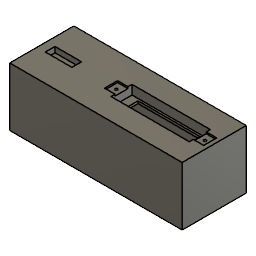
Base Pantalla - Pila T.D.I (Autodesk Fusion 360 design; units mm, degrees)
part number: 2026-07-05-14-44-51-379
Autodesk Fusion 360 part; units mm, degrees
note: some values were not read from the file. Set by a fixed rule: which sketch regions a step uses.
sketch "Boceto1" plane through (0, 0, 0) normal (0, 1, 0) x (1, 0, 0)
  line L0 (0, 0) -> (220, 0)
  line L1 (220, 0) -> (220, 60)
  line L2 (220, 60) -> (0, 60)
  line L3 (0, 60) -> (0, 0)
  line L4 (227, -7) -> (227, 67)
  line L5 (227, 67) -> (-7, 67)
  line L6 (-7, 67) -> (-7, -7)
  line L7 (-7, -7) -> (227, -7)
  line L8 (217, 3) -> (217, 57)
  line L9 (217, 57) -> (3, 57)
  line L10 (3, 57) -> (3, 3)
  line L11 (3, 3) -> (217, 3)
  dimension "d1" = 220
  dimension "d2" = 60
  dimension "d3" = 7
  dimension "d4" = -3
  constraint horizontal L0
  constraint vertical L1
  constraint horizontal L2
  constraint vertical L3
  constraint coincident L0.start L3.end
  measures "d1" distance of L0.start L0.end
  measures "d2" distance of L0.start L2.end
extrude "Extruir1" add sketch "Boceto1" along normal blind 3 contours L4 L5 L6 L7
sketch "Boceto2" plane through (0, 0, 0) normal (0, 1, 0) x (1, 0, 0)
  line L0 (0, 0) -> (220, 0)
  line L1 (220, 0) -> (220, 60)
  line L2 (220, 60) -> (0, 60)
  line L3 (0, 60) -> (0, 0)
  line L4 (3, 3) -> (217, 3)
  line L5 (217, 3) -> (217, 57)
  line L6 (217, 57) -> (3, 57)
  line L7 (3, 57) -> (3, 3)
  dimension "d7" = -3
  constraint horizontal L0
  constraint vertical L1
  constraint horizontal L2
  constraint vertical L3
  constraint coincident L0.start L3.end
extrude "Extruir2" add sketch "Boceto2" along normal blind 40
sketch "Boceto3" plane through (0, 40, 0) normal (0, 1, 0) x (-1, 0, 0)
  line L0 (-3, -3) -> (-3, -57)
  line L1 (-3, -57) -> (-217, -57)
  line L2 (-217, -57) -> (-217, -3)
  line L3 (-217, -3) -> (-3, -3)
  line L4 (0, -60) -> (0, 0)
  line L5 (0, 0) -> (-220, 0)
  line L6 (-220, 0) -> (-220, -60)
  line L7 (-220, -60) -> (0, -60)
  line L8 (0, 0) -> (-220, 0)
  line L9 (-220, 0) -> (-220, -60)
  line L10 (-220, -60) -> (0, -60)
  line L11 (0, -60) -> (0, 0)
  line L12 (0, 0) -> (-220, 0)
  line L13 (-220, 0) -> (-220, -60)
  line L14 (-220, -60) -> (0, -60)
  line L15 (0, -60) -> (0, 0)
  constraint horizontal L8
  constraint vertical L9
  constraint horizontal L10
  constraint vertical L11
  constraint coincident L6.end L7.start
  constraint coincident L4.end L5.start
  constraint horizontal L12
  constraint vertical L13
  constraint horizontal L14
  constraint vertical L15
extrude "Extruir3" add sketch "Boceto3" along normal blind 3 contours L0 L1 L2 L3 | L4 L5 L6 L7 L8 L9 L10 L11 L12 L13 L14 L15
sketch "Boceto4" plane through (0, 43, 0) normal (0, 1, 0) x (-1, 0, 0)
  line L0 (0, -60) -> (0, 0)
  line L1 (0, 0) -> (-220, 0)
  line L2 (-220, 0) -> (-220, -60)
  line L3 (-220, -60) -> (0, -60)
  line L4 (-25, -35.99) -> (-53.57, -35.99)
  line L5 (-53.57, -35.99) -> (-53.57, -24.01)
  line L6 (-53.57, -24.01) -> (-25, -24.01)
  line L7 (-25, -24.01) -> (-25, -35.99)
  dimension "d15" = 28.57
  dimension "d16" = 11.98
  constraint horizontal L4
  constraint vertical L5
  constraint horizontal L6
  constraint vertical L7
  measures "d15" distance of L4.start L4.end
  measures "d16" distance of L4.start L6.end
extrude "Extruir4" cut sketch "Boceto4" against normal blind 3 contours L4 L5 L6 L7
sketch "Boceto5" plane through (0, 43, 0) normal (0, 1, 0) x (-1, 0, 0)
  line L0 (-53.57, -35.99) -> (-53.57, -24.01)
  line L1 (-53.57, -24.01) -> (-25, -24.01)
  line L2 (-25, -24.01) -> (-25, -35.99)
  line L3 (-25, -35.99) -> (-53.57, -35.99)
  line L4 (0, -60) -> (0, 0)
  line L5 (0, 0) -> (-220, 0)
  line L6 (-220, 0) -> (-220, -60)
  line L7 (-220, -60) -> (0, -60)
  line L8 (-197, -40.593) -> (-119.4, -40.593)
  line L9 (-119.4, -40.593) -> (-119.4, -19.407)
  line L10 (-119.4, -19.407) -> (-197, -19.407)
  line L11 (-197, -19.407) -> (-197, -40.593)
  point P0 (-220, -30)
  point P1 (-197, -40.593)
  dimension "d22" = 77.6
  dimension "d23" = 21.186
  constraint horizontal L8
  constraint vertical L9
  constraint horizontal L10
  constraint vertical L11
  constraint coincident P1 L8.start
  measures "d22" distance of P1 L8.end
  measures "d23" distance of P1 L10.end
extrude "Extruir5" cut sketch "Boceto5" against normal blind 3 contours L8 L9 L10 L11
sketch "Boceto6" plane through (0, 40, 0) normal (0, -1, 0) x (1, 0, 0)
  line L0 (197, -40.593) -> (119.4, -40.593)
  line L1 (119.4, -40.593) -> (119.4, -19.407)
  line L2 (119.4, -19.407) -> (197, -19.407)
  line L3 (197, -19.407) -> (197, -40.593)
  line L4 (53.57, -24.01) -> (53.57, -35.99)
  line L5 (53.57, -35.99) -> (25, -35.99)
  line L6 (25, -35.99) -> (25, -24.01)
  line L7 (25, -24.01) -> (53.57, -24.01)
  line L8 (217, -3) -> (3, -3)
  line L9 (3, -3) -> (3, -57)
  line L10 (3, -57) -> (217, -57)
  line L11 (217, -57) -> (217, -3)
  line L12 (200, -43.593) -> (116.4, -43.593)
  line L13 (116.4, -43.593) -> (116.4, -16.407)
  line L14 (116.4, -16.407) -> (200, -16.407)
  line L15 (200, -16.407) -> (200, -43.593)
  dimension "d26" = -3
extrude "Extruir6" add sketch "Boceto6" along normal blind 11.5 contours L12 L13 L14 L15
sketch "Boceto7" plane through (0, 43, 0) normal (0, 1, 0) x (-1, 0, 0)
  line L0 (-119.4, -40.593) -> (-197, -40.593)
  line L1 (-197, -40.593) -> (-197, -19.407)
  line L2 (-197, -19.407) -> (-119.4, -19.407)
  line L3 (-119.4, -19.407) -> (-119.4, -40.593)
  line L4 (-53.57, -35.99) -> (-53.57, -24.01)
  line L5 (-53.57, -24.01) -> (-25, -24.01)
  line L6 (-25, -24.01) -> (-25, -35.99)
  line L7 (-25, -35.99) -> (-53.57, -35.99)
  line L8 (0, -60) -> (0, 0)
  line L9 (0, 0) -> (-220, 0)
  line L10 (-220, 0) -> (-220, -60)
  line L11 (-220, -60) -> (0, -60)
  line L12 (0, 0) -> (-220, 0)
  line L13 (-220, 0) -> (-220, -60)
  line L14 (-220, -60) -> (0, -60)
  line L15 (0, -60) -> (0, 0)
  line L16 (-230, -70) -> (10, -70)
  line L17 (10, -70) -> (10, 10)
  line L18 (10, 10) -> (-230, 10)
  line L19 (-230, 10) -> (-230, -70)
  dimension "d29" = 10
  constraint horizontal L12
  constraint vertical L13
  constraint horizontal L14
  constraint vertical L15
  constraint coincident L10.end L11.start
  constraint coincident L8.end L9.start
extrude "Extruir7" add sketch "Boceto7" against normal blind 43 contours L16 L17 L18 L19
sketch "Boceto8" plane through (0, 43, 0) normal (0, 1, 0) x (-1, 0, 0)
  line L0 (-230, 10) -> (-230, -70)
  line L1 (-230, -70) -> (10, -70)
  line L2 (10, -70) -> (10, 10)
  line L3 (10, 10) -> (-230, 10)
  line L4 (-119.4, -40.593) -> (-197, -40.593)
  line L5 (-197, -40.593) -> (-197, -19.407)
  line L6 (-197, -19.407) -> (-119.4, -19.407)
  line L7 (-119.4, -19.407) -> (-119.4, -40.593)
  line L8 (-53.57, -35.99) -> (-53.57, -24.01)
  line L9 (-53.57, -24.01) -> (-25, -24.01)
  line L10 (-25, -24.01) -> (-25, -35.99)
  line L11 (-25, -35.99) -> (-53.57, -35.99)
sketch "Boceto9" plane through (0, 0, 0) normal (0, -1, 0) x (1, 0, 0)
  line L0 (230, -70) -> (230, 10)
  line L1 (230, 10) -> (-10, 10)
  line L2 (-10, 10) -> (-10, -70)
  line L3 (-10, -70) -> (230, -70)
  line L4 (3, -57) -> (3, -3)
  line L5 (3, -3) -> (217, -3)
  line L6 (217, -3) -> (217, -57)
  line L7 (217, -57) -> (3, -57)
  line L8 (-10, 10) -> (-7, 10)
  line L9 (-7, 10) -> (-7, 7)
  line L10 (-7, 7) -> (-10, 7)
  line L11 (-10, 7) -> (-10, 10)
  line L12 (230, -70) -> (227, -70)
  line L13 (227, -70) -> (227, -67)
  line L14 (227, -67) -> (230, -67)
  line L15 (230, -67) -> (230, -70)
  line L16 (-7, 7) -> (227, 7)
  line L17 (227, 7) -> (227, -67)
  line L18 (227, -67) -> (-7, -67)
  line L19 (-7, -67) -> (-7, 7)
  dimension "d32" = 3
  dimension "d33" = 3
  dimension "d34" = 3
  dimension "d35" = 3
  constraint horizontal L8
  constraint vertical L9
  constraint horizontal L10
  constraint vertical L11
  constraint coincident L1.end L2.start
  constraint horizontal L12
  constraint vertical L13
  constraint horizontal L14
  constraint vertical L15
  constraint coincident L0.start L3.end
  constraint horizontal L16
  constraint vertical L17
  constraint horizontal L18
  constraint vertical L19
  measures "d32" distance of L1.end L8.end
  measures "d33" distance of L1.end L10.end
  measures "d34" distance of L0.start L12.end
  measures "d35" distance of L0.start L14.end
extrude "Extruir8" cut sketch "Boceto9" against normal blind 40 contours L16 L17 L18 L19
sketch "Boceto10" plane through (0, 40, 0) normal (0, -1, 0) x (1, 0, 0)
  line L0 (-7, -67) -> (227, -67)
  line L1 (227, -67) -> (227, 7)
  line L2 (227, 7) -> (-7, 7)
  line L3 (-7, 7) -> (-7, -67)
  line L4 (200, -16.407) -> (200, -43.593)
  line L5 (200, -43.593) -> (116.4, -43.593)
  line L6 (116.4, -43.593) -> (116.4, -16.407)
  line L7 (116.4, -16.407) -> (200, -16.407)
  line L8 (53.57, -24.01) -> (53.57, -35.99)
  line L9 (53.57, -35.99) -> (25, -35.99)
  line L10 (25, -35.99) -> (25, -24.01)
  line L11 (25, -24.01) -> (53.57, -24.01)
  line L12 (56.57, -38.99) -> (22, -38.99)
  line L13 (22, -38.99) -> (22, -21.01)
  line L14 (22, -21.01) -> (56.57, -21.01)
  line L15 (56.57, -21.01) -> (56.57, -38.99)
  dimension "d38" = -3
extrude "Extruir9" add sketch "Boceto10" along normal blind 3.8 contours L12 L13 L14 L15
sketch "Boceto11" plane through (0, 36.2, 0) normal (0, -1, 0) x (1, 0, 0)
  line L0 (25, -35.99) -> (25, -24.01)
  line L1 (25, -24.01) -> (53.57, -24.01)
  line L2 (53.57, -24.01) -> (53.57, -35.99)
  line L3 (53.57, -35.99) -> (25, -35.99)
  line L4 (56.57, -21.01) -> (22, -21.01)
  line L5 (22, -21.01) -> (22, -38.99)
  line L6 (22, -38.99) -> (56.57, -38.99)
  line L7 (56.57, -38.99) -> (56.57, -21.01)
  line L8 (22, -21.01) -> (56.57, -21.01)
  line L9 (56.57, -21.01) -> (56.57, -38.99)
  line L10 (56.57, -38.99) -> (22, -38.99)
  line L11 (22, -38.99) -> (22, -21.01)
  constraint horizontal L8
  constraint vertical L9
  constraint horizontal L10
  constraint vertical L11
  constraint coincident L6.end L7.start
  constraint coincident L4.end L5.start
extrude "Extruir10" add sketch "Boceto11" along normal blind 3 contours L0 L1 L2 L3 | L4 L5 L6 L7 L8 L9 L10 L11
sketch "Boceto12" plane through (56.57, 0, 0) normal (1, 0, 0) x (0, 0, -1)
  line L0 (38.99, 40) -> (21.01, 40)
  line L1 (21.01, 40) -> (21.01, 33.2)
  line L2 (21.01, 33.2) -> (38.99, 33.2)
  line L3 (38.99, 33.2) -> (38.99, 40)
  line L4 (21.01, 40) -> (24.01, 40)
  line L5 (38.99, 40) -> (35.99, 40)
  line L6 (24.01, 40) -> (35.99, 40)
  line L7 (35.99, 40) -> (35.99, 36.2)
  line L8 (35.99, 36.2) -> (24.01, 36.2)
  line L9 (24.01, 36.2) -> (24.01, 40)
  dimension "d43" = 3
  dimension "d44" = 3
  dimension "d45" = 11.98
  dimension "d46" = 3.8
  constraint coincident L0.end L1.start
  constraint perpendicular L1 L4
  constraint coincident L0.start L3.end
  constraint perpendicular L3 L5
  constraint horizontal L6
  constraint vertical L7
  constraint horizontal L8
  constraint vertical L9
  measures "d43" distance of L0.end L4.end
  measures "d44" distance of L0.start L5.end
  measures "d45" distance of L4.end L5.end
  measures "d46" distance of L4.end L8.end
extrude "Extruir11" cut sketch "Boceto12" against normal blind 3 contours L0 L6 L7 L8 L9
sketch "Boceto13" plane through (56.57, 0, 0) normal (1, 0, 0) x (0, 0, -1)
  line L0 (24.01, 36.2) -> (24.01, 40)
  line L1 (24.01, 40) -> (21.01, 40)
  line L2 (21.01, 40) -> (21.01, 33.2)
  line L3 (21.01, 33.2) -> (38.99, 33.2)
  line L4 (38.99, 33.2) -> (38.99, 40)
  line L5 (38.99, 40) -> (35.99, 40)
  line L6 (35.99, 40) -> (35.99, 36.2)
  line L7 (35.99, 36.2) -> (24.01, 36.2)
  line L8 (21.01, 40) -> (38.99, 40)
  line L9 (38.99, 40) -> (38.99, 33.2)
  line L10 (38.99, 33.2) -> (21.01, 33.2)
  line L11 (21.01, 33.2) -> (21.01, 40)
  constraint horizontal L8
  constraint vertical L9
  constraint horizontal L10
  constraint vertical L11
  constraint coincident L3.end L4.start
  constraint coincident L1.end L2.start
extrude "Extruir12" cut sketch "Boceto13" against normal blind 3 contours L0 L1 L2 L3 L4 L5 L6 L7 L8 L9 L10 L11
sketch "Boceto14" plane through (25, 0, 0) normal (1, 0, 0) x (0, 0, -1)
  line L0 (35.99, 43) -> (24.01, 43)
  line L1 (24.01, 43) -> (24.01, 36.2)
  line L2 (24.01, 36.2) -> (35.99, 36.2)
  line L3 (35.99, 36.2) -> (35.99, 43)
  line L4 (24.01, 43) -> (35.99, 43)
  line L5 (35.99, 43) -> (35.99, 36.2)
  line L6 (35.99, 36.2) -> (24.01, 36.2)
  line L7 (24.01, 36.2) -> (24.01, 43)
  constraint horizontal L4
  constraint vertical L5
  constraint horizontal L6
  constraint vertical L7
  constraint coincident L2.end L3.start
  constraint coincident L0.end L1.start
extrude "Extruir13" add sketch "Boceto14" against normal blind 4.56
extrude "Extruir14" add 1 faces at (22, 34.2, -28.0033) along direction (-1, 0, 0) blind 4.56
extrude "Extruir15" cut 1 faces at (25, 40.7333, -31.9967) along direction (-1, 0, 0) blind 4.56
sketch "Boceto15" plane through (17.44, 0, 0) normal (-1, 0, 0) x (0, 0, 1)
  line L0 (-35.99, 36.2) -> (-35.99, 40)
  line L1 (-35.99, 40) -> (-38.99, 40)
  line L2 (-38.99, 40) -> (-38.99, 33.2)
  line L3 (-38.99, 33.2) -> (-21.01, 33.2)
  line L4 (-21.01, 33.2) -> (-21.01, 40)
  line L5 (-21.01, 40) -> (-24.01, 40)
  line L6 (-24.01, 40) -> (-24.01, 36.2)
  line L7 (-24.01, 36.2) -> (-35.99, 36.2)
  line L8 (-38.99, 33.2) -> (-21.01, 33.2)
  line L9 (-21.01, 33.2) -> (-21.01, 40)
  line L10 (-21.01, 40) -> (-38.99, 40)
  line L11 (-38.99, 40) -> (-38.99, 33.2)
  constraint horizontal L8
  constraint vertical L9
  constraint horizontal L10
  constraint vertical L11
  constraint coincident L4.end L5.start
  constraint coincident L2.end L3.start
extrude "Extruir16" add sketch "Boceto15" against normal blind 3 contours L0 L6 L7 L10
sketch "Boceto16" plane through (0, 0, 0) normal (0, -1, 0) x (1, 0, 0)
  line L0 (227, 7) -> (227, -67)
  line L1 (227, -67) -> (-7, -67)
  line L2 (-7, -67) -> (-7, 7)
  line L3 (-7, 7) -> (227, 7)
  line L4 (230, -70) -> (230, 10)
  line L5 (230, 10) -> (-10, 10)
  line L6 (-10, 10) -> (-10, -70)
  line L7 (-10, -70) -> (230, -70)
  line L8 (230, 10) -> (245, 10)
  line L9 (245, 10) -> (245, -70)
  line L10 (245, -70) -> (230, -70)
  line L11 (230, -70) -> (230, 10)
  line L12 (-10, 10) -> (-25, 10)
  line L13 (-25, 10) -> (-25, -70)
  line L14 (-25, -70) -> (-10, -70)
  line L15 (-10, -70) -> (-10, 10)
  dimension "d59" = 15
  dimension "d60" = 80
  dimension "d61" = 15
  dimension "d62" = 80
  constraint horizontal L8
  constraint vertical L9
  constraint horizontal L10
  constraint vertical L11
  constraint coincident L4.end L5.start
  constraint horizontal L12
  constraint vertical L13
  constraint horizontal L14
  constraint vertical L15
  constraint coincident L5.end L6.start
  measures "d59" distance of L4.end L8.end
  measures "d60" distance of L4.end L4.start
  measures "d61" distance of L5.end L12.end
  measures "d62" distance of L5.end L6.end
extrude "Extruir17" add sketch "Boceto16" against normal blind 3 contours L4 L8 L9 L10 L11 | L6 L12 L13 L14 L15
sketch "Boceto17" plane through (0, 3, 0) normal (0, 1, 0) x (-1, 0, 0)
  line L0 (10, 10) -> (10, -70)
  line L1 (10, -70) -> (25, -70)
  line L2 (25, -70) -> (25, 10)
  line L3 (25, 10) -> (10, 10)
  circle A0 centre (17.5, 1.5623) radius 3.375
  circle A1 centre (16.8728, -62.4918) radius 3.375
  circle A2 centre (-237.4689, -62.1794) radius 3.375
  circle A3 centre (-237.1564, 2.4997) radius 3.375
  dimension "d65" = 6.75
  dimension "d66" = 6.75
  dimension "d67" = 6.75
  dimension "d68" = 6.75
  measures "d65" diameter of A0
  measures "d66" diameter of A1
  measures "d67" diameter of A2
  measures "d68" diameter of A3
extrude "Extruir18" cut sketch "Boceto17" against normal blind 3 contours A0 | A1 | A2 | A3
sketch "Boceto18" plane through (0, 0, 0) normal (0, -1, 0) x (1, 0, 0)
  line L0 (245, 10) -> (-25, 10)
  line L1 (-25, 10) -> (-25, -70)
  line L2 (-25, -70) -> (245, -70)
  line L3 (245, -70) -> (245, 10)
  line L4 (227, 7) -> (227, -67)
  line L5 (227, -67) -> (-7, -67)
  line L6 (-7, -67) -> (-7, 7)
  line L7 (-7, 7) -> (227, 7)
  circle A0 centre (237.4689, -62.1794) radius 3.375
  circle A1 centre (-16.8728, -62.4918) radius 3.375
  circle A2 centre (237.1564, 2.4997) radius 3.375
  circle A3 centre (-17.5, 1.5623) radius 3.375
  line L8 (-25, 10) -> (245, 10)
  line L9 (245, 10) -> (245, -70)
  line L10 (245, -70) -> (-25, -70)
  line L11 (-25, -70) -> (-25, 10)
  constraint horizontal L8
  constraint vertical L9
  constraint horizontal L10
  constraint vertical L11
  constraint coincident L2.end L3.start
  constraint coincident L0.end L1.start
extrude "Extruir19" add sketch "Boceto18" along normal blind 30
sketch "Boceto19" plane through (0, 3, 0) normal (0, 1, 0) x (-1, 0, 0)
  circle A0 centre (17.5, 1.5623) radius 3.375
  circle A1 centre (16.8728, -62.4918) radius 3.375
  line L0 (10, 10) -> (10, -70)
  line L1 (10, -70) -> (25, -70)
  line L2 (25, -70) -> (25, 10)
  line L3 (25, 10) -> (10, 10)
  line L4 (25, -70) -> (10, -70)
  line L5 (10, -70) -> (10, 10)
  line L6 (10, 10) -> (25, 10)
  line L7 (25, 10) -> (25, -70)
  line L8 (-230, -70) -> (-245, -70)
  line L9 (-245, -70) -> (-245, 10)
  line L10 (-245, 10) -> (-230, 10)
  line L11 (-230, 10) -> (-230, -70)
  constraint horizontal L4
  constraint vertical L5
  constraint horizontal L6
  constraint vertical L7
  constraint coincident L0.start L3.end
  constraint coincident L1.end L2.start
  constraint horizontal L8
  constraint vertical L9
  constraint horizontal L10
  constraint vertical L11
extrude "Extruir20" cut sketch "Boceto19" against normal blind 25
sketch "Boceto20" plane through (0, 43, 0) normal (0, 1, 0) x (-1, 0, 0)
  line L0 (-230, 10) -> (-230, -70)
  line L1 (-230, -70) -> (10, -70)
  line L2 (10, -70) -> (10, 10)
  line L3 (10, 10) -> (-230, 10)
  line L4 (-119.4, -40.593) -> (-197, -40.593)
  line L5 (-197, -40.593) -> (-197, -19.407)
  line L6 (-197, -19.407) -> (-119.4, -19.407)
  line L7 (-119.4, -19.407) -> (-119.4, -40.593)
  line L8 (-53.57, -24.01) -> (-20.44, -24.01)
  line L9 (-20.44, -24.01) -> (-20.44, -35.99)
  line L10 (-20.44, -35.99) -> (-53.57, -35.99)
  line L11 (-53.57, -35.99) -> (-53.57, -24.01)
  line L12 (-197, -19.407) -> (-119.4, -19.407)
  line L13 (-119.4, -19.407) -> (-119.4, -40.593)
  line L14 (-119.4, -40.593) -> (-197, -40.593)
  line L15 (-197, -40.593) -> (-197, -19.407)
  line L16 (-207, -50.593) -> (-207, -9.407)
  line L17 (-207, -9.407) -> (-109.4, -9.407)
  line L18 (-109.4, -9.407) -> (-109.4, -50.593)
  line L19 (-109.4, -50.593) -> (-207, -50.593)
  dimension "d75" = -10
  constraint horizontal L12
  constraint vertical L13
  constraint horizontal L14
  constraint vertical L15
  constraint coincident L4.start L7.end
  constraint coincident L5.end L6.start
extrude "Extruir21" add sketch "Boceto20" against normal blind 14.5 contours L16 L17 L18 L19
sketch "Boceto21" plane through (0, 28.5, 0) normal (0, -1, 0) x (1, 0, 0)
  line L0 (109.4, -9.407) -> (109.4, -50.593)
  line L1 (109.4, -50.593) -> (207, -50.593)
  line L2 (207, -50.593) -> (207, -9.407)
  line L3 (207, -9.407) -> (109.4, -9.407)
  line L4 (119.4, -19.407) -> (197, -19.407)
  line L5 (197, -19.407) -> (197, -40.593)
  line L6 (197, -40.593) -> (119.4, -40.593)
  line L7 (119.4, -40.593) -> (119.4, -19.407)
  line L8 (207, -50.593) -> (109.4, -50.593)
  line L9 (109.4, -50.593) -> (109.4, -9.407)
  line L10 (109.4, -9.407) -> (207, -9.407)
  line L11 (207, -9.407) -> (207, -50.593)
  line L12 (210, -6.407) -> (210, -53.593)
  line L13 (210, -53.593) -> (106.4, -53.593)
  line L14 (106.4, -53.593) -> (106.4, -6.407)
  line L15 (106.4, -6.407) -> (210, -6.407)
  dimension "d78" = -3
  constraint horizontal L8
  constraint vertical L9
  constraint horizontal L10
  constraint vertical L11
  constraint coincident L0.start L3.end
  constraint coincident L1.end L2.start
extrude "Extruir22" add sketch "Boceto21" against normal blind 11.5 contours L12 L13 L14 L15
sketch "Boceto22" plane through (0, 43, 0) normal (0, 1, 0) x (-1, 0, 0)
  line L0 (-119.4, -40.593) -> (-197, -40.593)
  line L1 (-197, -40.593) -> (-197, -19.407)
  line L2 (-197, -19.407) -> (-119.4, -19.407)
  line L3 (-119.4, -19.407) -> (-119.4, -40.593)
  line L4 (-230, 10) -> (-230, -70)
  line L5 (-230, -70) -> (10, -70)
  line L6 (10, -70) -> (10, 10)
  line L7 (10, 10) -> (-230, 10)
  line L8 (-53.57, -24.01) -> (-20.44, -24.01)
  line L9 (-20.44, -24.01) -> (-20.44, -35.99)
  line L10 (-20.44, -35.99) -> (-53.57, -35.99)
  line L11 (-53.57, -35.99) -> (-53.57, -24.01)
  line L12 (-197, -19.407) -> (-119.4, -19.407)
  line L13 (-119.4, -19.407) -> (-119.4, -40.593)
  line L14 (-119.4, -40.593) -> (-197, -40.593)
  line L15 (-197, -40.593) -> (-197, -19.407)
  line L16 (-207, -50.593) -> (-207, -9.407)
  line L17 (-207, -9.407) -> (-109.4, -9.407)
  line L18 (-109.4, -9.407) -> (-109.4, -50.593)
  line L19 (-109.4, -50.593) -> (-207, -50.593)
  dimension "d81" = -10
  constraint horizontal L12
  constraint vertical L13
  constraint horizontal L14
  constraint vertical L15
  constraint coincident L0.start L3.end
  constraint coincident L1.end L2.start
extrude "Extruir23" cut sketch "Boceto22" against normal blind 11.5 contours L16 L17 L18 L19
extrude "Extruir24" add 1 faces at (174.4667, 39.1667, -9.407) along direction (0, 0, -1) blind 7.5
extrude "Extruir25" add 1 faces at (141.9333, 39.1667, -50.593) along direction (0, 0, 1) blind 7.5
extrude "Extruir26" add 1 faces at (106.4, 32.3333, -37.8643) along direction (-1, 0, 0) blind 10
extrude "Extruir27" add 1 faces at (210, 32.3333, -22.1357) along direction (1, 0, 0) blind 17
sketch "Boceto23" plane through (0, 28.5, 0) normal (0, -1, 0) x (1, 0, 0)
  line L0 (96.4, -53.593) -> (227, -53.593)
  line L1 (227, -53.593) -> (227, -6.407)
  line L2 (227, -6.407) -> (96.4, -6.407)
  line L3 (96.4, -6.407) -> (96.4, -53.593)
  line L4 (119.4, -19.407) -> (197, -19.407)
  line L5 (197, -19.407) -> (197, -40.593)
  line L6 (197, -40.593) -> (119.4, -40.593)
  line L7 (119.4, -40.593) -> (119.4, -19.407)
  line L8 (96.4, -29.997) -> (227, -30)
  circle A0 centre (101.1931, -29.997) radius 3.375
  circle A1 centre (214.3398, -29.9985) radius 3.375
  dimension "d93" = 6.75
  dimension "d94" = 6.75
  constraint midpoint L1 L8.end
  measures "d93" diameter of A0
  measures "d94" diameter of A1
extrude "Extruir28" cut sketch "Boceto23" against normal blind 14.5 contours L8 A0 | L8 A0 | L8 A1 | L8 A1
sketch "Boceto24" plane through (0, 43, 0) normal (0, 1, 0) x (-1, 0, 0)
  circle A0 centre (-214.3398, -29.9985) radius 3.375
  circle A1 centre (-101.1931, -29.997) radius 3.375
  line L0 (-109.4, -16.907) -> (-109.4, -43.093)
  line L1 (-109.4, -43.093) -> (-207, -43.093)
  line L2 (-207, -43.093) -> (-207, -16.907)
  line L3 (-207, -16.907) -> (-109.4, -16.907)
  line L4 (-230, 10) -> (-230, -70)
  line L5 (-230, -70) -> (10, -70)
  line L6 (10, -70) -> (10, 10)
  line L7 (10, 10) -> (-230, 10)
  line L8 (-53.57, -24.01) -> (-20.44, -24.01)
  line L9 (-20.44, -24.01) -> (-20.44, -35.99)
  line L10 (-20.44, -35.99) -> (-53.57, -35.99)
  line L11 (-53.57, -35.99) -> (-53.57, -24.01)
  line L12 (-207, -16.907) -> (-207, -22.407)
  line L13 (-207, -22.407) -> (-220.2736, -22.407)
  line L14 (-220.2736, -22.407) -> (-220.2736, -37.593)
  line L15 (-220.2736, -37.593) -> (-207, -37.593)
  line L16 (-207, -37.593) -> (-207, -22.407)
  dimension "d98" = 5.5
  dimension "d99" = 15.186
  constraint coincident L2.end L3.start
  constraint perpendicular L1 L12
  constraint horizontal L13
  constraint vertical L14
  constraint horizontal L15
  constraint vertical L16
  measures "d98" distance of L2.end L12.end
  measures "d99" distance of L12.end L15.end
extrude "Extruir29" cut sketch "Boceto24" against normal blind 3 contours L2 L13 L14 L15 L16
sketch "Boceto25" plane through (0, 43, 0) normal (0, 1, 0) x (-1, 0, 0)
  line L0 (-220.2736, -22.407) -> (-207, -22.407)
  line L1 (-207, -22.407) -> (-207, -16.907)
  line L2 (-207, -16.907) -> (-109.4, -16.907)
  line L3 (-109.4, -16.907) -> (-109.4, -43.093)
  line L4 (-109.4, -43.093) -> (-207, -43.093)
  line L5 (-207, -43.093) -> (-207, -37.593)
  line L6 (-207, -37.593) -> (-220.2736, -37.593)
  line L7 (-220.2736, -37.593) -> (-220.2736, -22.407)
  circle A0 centre (-101.1931, -29.997) radius 3.375
  line L8 (-230, 10) -> (-230, -70)
  line L9 (-230, -70) -> (10, -70)
  line L10 (10, -70) -> (10, 10)
  line L11 (10, 10) -> (-230, 10)
  line L12 (-53.57, -24.01) -> (-20.44, -24.01)
  line L13 (-20.44, -24.01) -> (-20.44, -35.99)
  line L14 (-20.44, -35.99) -> (-53.57, -35.99)
  line L15 (-53.57, -35.99) -> (-53.57, -24.01)
  line L16 (-207, -22.407) -> (-85.5036, -22.407)
  line L17 (-109.4, -22.407) -> (-96.126, -22.407)
  line L18 (-96.126, -22.407) -> (-96.126, -37.593)
  line L19 (-96.126, -37.593) -> (-109.4, -37.593)
  line L20 (-109.4, -37.593) -> (-109.4, -22.407)
  dimension "d102" = 13.274
  dimension "d103" = 15.186
  constraint coincident L0.end L1.start
  constraint perpendicular L1 L16
  constraint horizontal L17
  constraint vertical L18
  constraint horizontal L19
  constraint vertical L20
  constraint coincident L16 L17.start
  constraint coincident L3 L17.start
  measures "d102" distance of L17.start L17.end
  measures "d103" distance of L17.start L19.end
extrude "Extruir30" cut sketch "Boceto25" against normal blind 3 contours L3 L16 L17 L18 L19 L20
extrude "Extruir31" add 1 faces at (96.4, 32.3333, -32.531) along direction (-1, 0, 0) blind 5
extrude "Extruir32" cut 1 faces at (96.126, 42, -27.469) along direction (-1, 0, 0) blind 1
sketch "Boceto26" plane through (0, 28.5, 0) normal (0, -1, 0) x (1, 0, 0)
  circle A0 centre (214.3398, -29.9985) radius 3.375
  circle A1 centre (101.1931, -29.997) radius 3.375
  line L0 (91.4, -53.593) -> (227, -53.593)
  line L1 (227, -53.593) -> (227, -6.407)
  line L2 (227, -6.407) -> (91.4, -6.407)
  line L3 (91.4, -6.407) -> (91.4, -53.593)
  line L4 (119.4, -19.407) -> (197, -19.407)
  line L5 (197, -19.407) -> (197, -40.593)
  line L6 (197, -40.593) -> (119.4, -40.593)
  line L7 (119.4, -40.593) -> (119.4, -19.407)
  line L8 (96.7391, -25.3343) -> (105, -25.3343)
  line L9 (105, -25.3343) -> (105, -35)
  line L10 (105, -35) -> (96.7391, -35)
  line L11 (96.7391, -35) -> (96.7391, -25.3343)
  line L12 (210.0534, -25.3343) -> (218.8583, -25.3343)
  line L13 (218.8583, -25.3343) -> (218.8583, -33.797)
  line L14 (218.8583, -33.797) -> (210.0534, -33.797)
  line L15 (210.0534, -33.797) -> (210.0534, -25.3343)
  constraint horizontal L8
  constraint vertical L9
  constraint horizontal L10
  constraint vertical L11
  constraint horizontal L12
  constraint vertical L13
  constraint horizontal L14
  constraint vertical L15
extrude "Extruir33" add sketch "Boceto26" against normal blind 7 contours A0 | A1 | L8 L9 L10 L11 | L12 L13 L14 L15
sketch "Boceto27" plane through (0, 43, 0) normal (0, 1, 0) x (-1, 0, 0)
  line L0 (-95.126, -37.593) -> (-109.4, -37.593)
  line L1 (-109.4, -37.593) -> (-109.4, -43.093)
  line L2 (-109.4, -43.093) -> (-207, -43.093)
  line L3 (-207, -43.093) -> (-207, -37.593)
  line L4 (-207, -37.593) -> (-220.2736, -37.593)
  line L5 (-220.2736, -37.593) -> (-220.2736, -22.407)
  line L6 (-220.2736, -22.407) -> (-207, -22.407)
  line L7 (-207, -22.407) -> (-207, -16.907)
  line L8 (-207, -16.907) -> (-109.4, -16.907)
  line L9 (-109.4, -16.907) -> (-109.4, -22.407)
  line L10 (-109.4, -22.407) -> (-95.126, -22.407)
  line L11 (-95.126, -22.407) -> (-95.126, -37.593)
  line L12 (-230, 10) -> (-230, -70)
  line L13 (-230, -70) -> (10, -70)
  line L14 (10, -70) -> (10, 10)
  line L15 (10, 10) -> (-230, 10)
  line L16 (-53.57, -24.01) -> (-20.44, -24.01)
  line L17 (-20.44, -24.01) -> (-20.44, -35.99)
  line L18 (-20.44, -35.99) -> (-53.57, -35.99)
  line L19 (-53.57, -35.99) -> (-53.57, -24.01)
  line L20 (-95.126, -37.593) -> (-109.4, -37.593)
  line L21 (-109.4, -37.593) -> (-109.4, -22.407)
  line L22 (-109.4, -22.407) -> (-95.126, -22.407)
  line L23 (-95.126, -22.407) -> (-95.126, -37.593)
  line L24 (-220.2736, -37.593) -> (-207, -37.593)
  line L25 (-207, -37.593) -> (-207, -22.407)
  line L26 (-207, -22.407) -> (-220.2736, -22.407)
  line L27 (-220.2736, -22.407) -> (-220.2736, -37.593)
  point P0 (-95.126, -37.593)
  point P1 (-109.4, -22.407)
  point P2 (-220.2736, -37.593)
  point P3 (-207, -22.407)
  constraint coincident P0 L0.start
  constraint coincident P1 L9.end
  constraint coincident P2 L4.end
  constraint coincident P3 L6.end
  constraint horizontal L20
  constraint vertical L21
  constraint horizontal L22
  constraint vertical L23
  constraint horizontal L24
  constraint vertical L25
  constraint horizontal L26
  constraint vertical L27
extrude "Extruir34" add sketch "Boceto27" against normal blind 3 contours L0 L10 L11 L20 L21 L22 L23 | L4 L5 L6 L24 L25 L26 L27
sketch "Boceto28" plane through (0, 43, 0) normal (0, 1, 0) x (-1, 0, 0)
  line L0 (-109.4, -16.907) -> (-109.4, -43.093)
  line L1 (-109.4, -43.093) -> (-207, -43.093)
  line L2 (-207, -43.093) -> (-207, -16.907)
  line L3 (-207, -16.907) -> (-109.4, -16.907)
  line L4 (-230, 10) -> (-230, -70)
  line L5 (-230, -70) -> (10, -70)
  line L6 (10, -70) -> (10, 10)
  line L7 (10, 10) -> (-230, 10)
  line L8 (-53.57, -24.01) -> (-20.44, -24.01)
  line L9 (-20.44, -24.01) -> (-20.44, -35.99)
  line L10 (-20.44, -35.99) -> (-53.57, -35.99)
  line L11 (-53.57, -35.99) -> (-53.57, -24.01)
  line L12 (-109.4, -43.093) -> (-109.4, -38.093)
  line L13 (-109.4, -38.093) -> (-96.4, -38.093)
  line L14 (-96.4, -38.093) -> (-96.4, -21.907)
  line L15 (-96.4, -21.907) -> (-109.4, -21.907)
  line L16 (-109.4, -21.907) -> (-109.4, -38.093)
  line L17 (-207, -43.093) -> (-207, -38.093)
  line L18 (-207, -38.093) -> (-220, -38.093)
  line L19 (-220, -38.093) -> (-220, -21.907)
  line L20 (-220, -21.907) -> (-207, -21.907)
  line L21 (-207, -21.907) -> (-207, -38.093)
  dimension "d114" = 5
  dimension "d115" = 13
  dimension "d116" = 16.186
  dimension "d117" = 5
  dimension "d118" = 13
  dimension "d119" = 16.186
  constraint coincident L0.end L1.start
  constraint perpendicular L1 L12
  constraint horizontal L13
  constraint vertical L14
  constraint horizontal L15
  constraint vertical L16
  constraint coincident L1.end L2.start
  constraint perpendicular L1 L17
  constraint horizontal L18
  constraint vertical L19
  constraint horizontal L20
  constraint vertical L21
  measures "d114" distance of L0.end L12.end
  measures "d115" distance of L12.end L13.end
  measures "d116" distance of L12.end L15.end
  measures "d117" distance of L1.end L17.end
  measures "d118" distance of L17.end L18.end
  measures "d119" distance of L17.end L20.end
extrude "Extruir35" cut sketch "Boceto28" against normal blind 5 contours L0 L13 L14 L15 L16 | L2 L18 L19 L20 L21
sketch "Boceto29" plane through (0, 38, 0) normal (0, 1, 0) x (-1, 0, 0)
  circle A0 centre (-101.1931, -29.997) radius 3.375
  line L0 (-109.4, -21.907) -> (-109.4, -38.093)
  line L1 (-109.4, -38.093) -> (-96.4, -38.093)
  line L2 (-96.4, -38.093) -> (-96.4, -21.907)
  line L3 (-96.4, -21.907) -> (-109.4, -21.907)
  line L4 (-109.4, -38.093) -> (-96.4, -38.093)
  line L5 (-96.4, -38.093) -> (-96.4, -21.907)
  line L6 (-96.4, -21.907) -> (-109.4, -21.907)
  line L7 (-109.4, -21.907) -> (-109.4, -38.093)
  constraint horizontal L4
  constraint vertical L5
  constraint horizontal L6
  constraint vertical L7
  constraint coincident L2.end L3.start
  constraint coincident L0.end L1.start
extrude "Extruir36" add 1 faces at (101.7722, 35.5, -28.9498) along direction (0, 1, 0) blind 2.5
extrude "Extruir37" add 1 faces at (212.977, 35.5, -30.9276) along direction (0, 1, 0) blind 2.5
sketch "Boceto30" plane through (0, 38, 0) normal (0, 1, 0) x (-1, 0, 0)
  line L0 (-109.4, -21.907) -> (-109.4, -38.093)
  line L1 (-109.4, -38.093) -> (-96.4, -38.093)
  line L2 (-96.4, -38.093) -> (-96.4, -21.907)
  line L3 (-96.4, -21.907) -> (-109.4, -21.907)
  line L4 (-109.4, -38.093) -> (-109.4, -30)
  line L5 (-109.4, -30) -> (-102.9, -30)
  circle A0 centre (-102.9, -30) radius 1.6
  dimension "d126" = 8.093
  dimension "d127" = 6.5
  dimension "d128" = 3.2
  constraint coincident L0.end L1.start
  constraint perpendicular L3 L4
  constraint perpendicular L2 L5
  constraint coincident L5.end A0.centre
  measures "d126" distance of L0.end L4.end
  measures "d127" distance of L4.end L5.end
  measures "d128" diameter of A0
extrude "Extruir38" cut sketch "Boceto30" against normal blind 3 contours A0
sketch "Boceto31" plane through (0, 38, 0) normal (0, 1, 0) x (-1, 0, 0)
  line L0 (-207, -21.907) -> (-220, -21.907)
  line L1 (-220, -21.907) -> (-220, -38.093)
  line L2 (-220, -38.093) -> (-207, -38.093)
  line L3 (-207, -38.093) -> (-207, -21.907)
  line L4 (-207, -38.093) -> (-207, -30)
  circle A0 centre (-213.5, -30) radius 1.6
  dimension "d133" = 3.2
  constraint coincident L2.end L3.start
  constraint perpendicular L0 L4
  measures "d133" diameter of A0
extrude "Extruir39" cut sketch "Boceto31" against normal blind 3 contours A0
extrude "Extruir40" add 1 faces at (102.9399, 38, -24.0728) along direction (0, 1, 0) blind 3
extrude "Extruir41" add 1 faces at (213.5399, 38, -24.0728) along direction (0, 1, 0) blind 3
extrude "Extruir42" add 1 faces at (103.1667, 35, -30.9247) along direction (0, 1, 0) blind 3
extrude "Extruir43" add 1 faces at (213.109, 35, -29.4783) along direction (0, 1, 0) blind 3
extrude "Extruir44" cut 1 faces at (-17.5841, -22, 8.3093) along direction (0, -1, 0) blind 7
extrude "Extruir45" cut 1 faces at (-17.5841, -29, 8.3093) along direction (0, -1, 0) blind 1
extrude "Extruir46" cut 1 faces at (243.5647, -22, -40.3949) along direction (0, -1, 0) blind 8
extrude "Extruir47" cut 1 faces at (-10, 18.6667, -16.6667) along direction (1, 0, 0) blind 10
sketch "Boceto32" plane through (0, 0, 0) normal (-1, 0, 0) x (0, 0, 1)
  line L0 (-67, -30) -> (-67, 40)
  line L1 (-67, 40) -> (7, 40)
  line L2 (7, 40) -> (7, -30)
  line L3 (7, -30) -> (10, -30)
  line L4 (10, -30) -> (10, 43)
  line L5 (10, 43) -> (-70, 43)
  line L6 (-70, 43) -> (-70, -30)
  line L7 (-70, -30) -> (-67, -30)
  line L8 (-70, 43) -> (10, 43)
  line L9 (10, 43) -> (10, -30)
  line L10 (10, -30) -> (-70, -30)
  line L11 (-70, -30) -> (-70, 43)
  constraint horizontal L8
  constraint vertical L9
  constraint horizontal L10
  constraint vertical L11
  constraint coincident L3.end L4.start
  constraint coincident L5.end L6.start
extrude "Extruir48" add sketch "Boceto32" against normal blind 3 contours L0 L1 L2 L10
extrude "Extruir49" cut 1 faces at (230, 18.6667, -16.6667) along direction (-1, 0, 0) blind 5
sketch "Boceto33" plane through (225, 0, 0) normal (1, 0, 0) x (0, 0, -1)
  line L0 (-7, -30) -> (-7, 40)
  line L1 (-7, 40) -> (6.407, 40)
  line L2 (6.407, 40) -> (6.407, 28.5)
  line L3 (6.407, 28.5) -> (53.593, 28.5)
  line L4 (53.593, 28.5) -> (53.593, 40)
  line L5 (53.593, 40) -> (67, 40)
  line L6 (67, 40) -> (67, -30)
  line L7 (67, -30) -> (70, -30)
  line L8 (70, -30) -> (70, 43)
  line L9 (70, 43) -> (-10, 43)
  line L10 (-10, 43) -> (-10, -30)
  line L11 (-10, -30) -> (-7, -30)
  line L12 (-10, 43) -> (70, 43)
  line L13 (70, 43) -> (70, -30)
  line L14 (70, -30) -> (-10, -30)
  line L15 (-10, -30) -> (-10, 43)
  constraint horizontal L12
  constraint vertical L13
  constraint horizontal L14
  constraint vertical L15
  constraint coincident L7.end L8.start
  constraint coincident L9.end L10.start
extrude "Extruir50" add sketch "Boceto33" against normal blind 3 contours L0 L1 L2 L3 L4 L5 L6 L14
extrude "Extruir51" cut 1 faces at (0, -5.6667, -16.6667) along direction (1, 0, 0) blind 10
sketch "Boceto34" plane through (10, 0, 0) normal (-1, 0, 0) x (0, 0, 1)
  line L0 (7, 40) -> (7, -30)
  line L1 (7, -30) -> (10, -30)
  line L2 (10, -30) -> (10, 43)
  line L3 (10, 43) -> (-70, 43)
  line L4 (-70, 43) -> (-70, -30)
  line L5 (-70, -30) -> (-67, -30)
  line L6 (-67, -30) -> (-67, 40)
  line L7 (-67, 40) -> (7, 40)
  line L8 (-70, 43) -> (10, 43)
  line L9 (10, 43) -> (10, -30)
  line L10 (10, -30) -> (-70, -30)
  line L11 (-70, -30) -> (-70, 43)
  constraint horizontal L8
  constraint vertical L9
  constraint horizontal L10
  constraint vertical L11
  constraint coincident L1.end L2.start
  constraint coincident L3.end L4.start
extrude "Extruir52" add sketch "Boceto34" against normal blind 3 contours L0 L6 L7 L10
equation "d46 = 6.8 mm - 3 mm"
equation "d53 = 4.56 mm - 3 mm + 3 mm"
equation "d99 = 20.686 mm - 5.5 mm"
equation "d116 = 21.186 mm - 5 mm"
equation "d119 = 21.186 mm - 5 mm"
equation "d126 = 16.186 * 0.5 mm"
equation "d127 = 13.000 * 0.5 mm"
equation "d136 = 5 mm - 2 mm"
equation "d138 = 5 mm - 2 mm"
equation "d140 = 6 mm - 3 mm"
equation "d142 = 6 mm - 3 mm"
